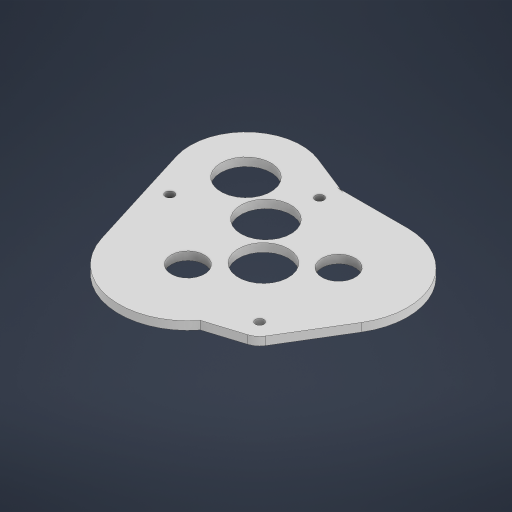
# Autodesk Inventor part: Part10
Saved by Autodesk Inventor 2024.4 (Build 284460000, 460)
## iProperties
Created: 2026-06-11
Part Number: Part10
Material: Generic
Document SubType Name: Modeling
Designer: stanr
Density: 1 g/cm^3
Appearance: Default
Author: stanr
Autodesk Inventor part; units mm, degrees
ref_plane "YZ Plane" through (0, 0, 0) normal (1, 0, 0) x (0, 1, 0)
ref_plane "XZ Plane" through (0, 0, 0) normal (0, 1, 0) x (-1, 0, 0)
ref_plane "XY Plane" through (0, 0, 0) normal (0, 0, 1) x (1, 0, 0)
sketch "Sketch2" plane through (0, 0, 0) normal (0, 1, 0) x (-1, 0, 0)
  circle A0 centre (0, 0) radius 22.86 construction
  circle A1 centre (20.8757, 22.3134) radius 9.525
  circle A2 centre (-23.8096, -19.1516) radius 9.525
  circle A3 centre (-23.8096, -19.1516) radius 25.4 construction
  circle A4 centre (-23.8096, -19.1516) radius 30.48 construction
  circle A5 centre (20.8757, 22.3134) radius 25.4 construction
  circle A6 centre (20.8757, 22.3134) radius 30.48 construction
  circle A7 centre (0, 0) radius 14.2875
  circle A8 centre (20.8757, -22.3134) radius 9.525 construction
  circle A9 centre (20.8757, 22.3134) radius 39.37
  circle A10 centre (-23.8096, -19.1516) radius 39.37
  circle A11 centre (20.8757, -22.3134) radius 14.2875
  circle A12 centre (-28.0225, 30.1989) radius 2.4892
  circle A13 centre (-28.0225, 30.1989) radius 6.35 construction
  line L0 (-21.7535, 29.1879) -> (-17.9921, 28.5813) construction
  line L1 (-27.4824, 23.8719) -> (-27.1583, 20.0757) construction
  circle A14 centre (16.2401, -48.2934) radius 2.4892
  circle A15 centre (16.2401, -48.2934) radius 6.35 construction
  line L2 (11.1056, -44.5573) -> (8.0248, -42.3156) construction
  circle A16 centre (47.4253, -37.4395) radius 22.86 construction
  line L3 (22.2373, -46.2061) -> (25.8356, -44.9537) construction
  circle A17 centre (60.6611, -7.1883) radius 2.4892
  circle A18 centre (60.6611, -7.1883) radius 6.35 construction
  line L4 (58.1157, -13.0059) -> (56.5885, -16.4964) construction
  line L5 (55.5604, -3.4061) -> (52.5, -1.1367) construction
  circle A19 centre (-28.0225, 30.1989) radius 10.16
  circle A20 centre (16.2401, -48.2934) radius 10.16
  circle A21 centre (60.6611, -7.1883) radius 10.16
  circle A22 centre (47.4253, -37.4395) radius 31.75
  line L6 (-57.4641, 1.278) -> (-36.7076, 35.471)
  line L7 (-10.2948, 46.3632) -> (-31.0445, 39.899)
  line L8 (58.4639, 34.0233) -> (70.3612, -4.1664)
  line L9 (77.7551, -28.05) -> (70.3666, -4.1837)
  circle A23 centre (47.4253, -37.4395) radius 14.2875
  line L10 (-23.7424, -58.5216) -> (16.2575, -58.4534)
  line L11 (12.4931, -57.7372) -> (35.7157, -66.9514)
  point P0 (16.2575, -58.4534)
  point P1 (13.1498, -5.587)
  point P2 (14.381, -9.5873)
  point P3 (15.7263, -35.6406)
  point P4 (15.6832, -38.1487)
  point P5 (8.0248, -42.3156)
  point P6 (12.6538, -33.9981)
  point P7 (8.5551, -15.0791)
  point P8 (4.5897, -13.5302)
  point P9 (14.3065, -58.4567)
  dimension "d0" = 45.72
  dimension "d2" = 19.05
  dimension "d3" = 50.8
  dimension "d4" = 60.96
  dimension "d5" = 30.5562
  dimension "d6" = 30.5562
  dimension "d7" = 28.575
  dimension "d8" = 30.5562
  dimension "d21" = 44.6853
  dimension "d22" = 8.89
  dimension "d23" = 8.89
  dimension "d25" = 4.9784
  dimension "d26" = 12.7
  dimension "d27" = 3.81
  dimension "d30" = 45.72
  dimension "d31" = 30.5562
  dimension "d32" = 65.3857
  dimension "d33" = 3.81
  dimension "d34" = 3.81
  dimension "d35" = 3.81
  dimension "d36" = 8.89
  dimension "d38" = 28.575
  dimension "d41" = 28.575
  constraints: 25 point on circle, 24 centre point, 24 end point, 12 point on line, 12 tangent, 10 coincident, 8 equal radius, 5 equal length, 1 perpendicular, 1 vertical alignment
  measures "d0" diameter of A0
  measures "d2" diameter of A2
  measures "d3" diameter of A3
  measures "d4" diameter of A4
  measures "d5" distance of A5.centre A0.centre
  measures "d6" distance of A2.centre point (0, 0)
  measures "d7" diameter of A7
  measures "d8" distance of point (0, 0) A8.centre
  measures "d21" horizontal distance of A2.centre A8.centre
  measures "d22" radial gap between concentric circles of A6 A9
  measures "d23" radial gap between concentric circles of A4 A10
  measures "d25" diameter of A12
  measures "d26" diameter of A13
  measures "d27" distance of L0.start L0.end
  measures "d30" diameter of A16
  measures "d31" distance of A8.centre A16.centre
  measures "d32" distance of A1.centre A16.centre
  measures "d33" radial gap between concentric circles of A13 A19
  measures "d34" radial gap between concentric circles of A15 A20
  measures "d35" radial gap between concentric circles of A18 A21
  measures "d36" radial gap between concentric circles of A16 A22
  measures "d38" diameter of A23
  measures "d41" diameter of A11
extrude "Extrusion1" add sketch "Sketch2" along normal blind 4.7625 contours A7 A10 A9 A22 A11 | A7 A9 A10 | A10 A11 A9 A7 | A7 A9 A11 A10 | A10 A19 A9 | A19 L7 A9 | A19 | A10 L6 A19 | A22 A9 A11 | A11 A22 A20 A10 | A9 A22 A21 A20 A11 | A9 A21 A22 | L8 A21 A9 | A10 A20 L11 L10 | A20 A22 A14 | A21 A22 A17 | A22 A17 A21 | L10 A20 A22 L11 | A20 A22 A14 | A21 L9 A22 picked at (-13.7968, 14.0826) picked at (38.7529, -8.9712)
equation "\"d6\" = d5"
equation "\"d8\" = d5"
body "Solid1"
